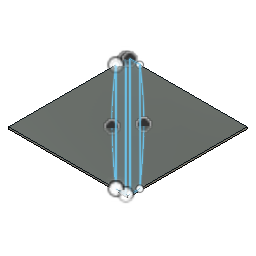
cnc2.2 (Autodesk Fusion 360 design; units mm, degrees)
Autodesk Fusion 360 part; units mm, degrees
sketch "Sketch1" plane through (0, 0, 0) normal (0, 0, 1) x (1, 0, 0)
  line L0 (-120, 100) -> (180, 100)
  line L1 (180, 100) -> (180, -200)
  line L2 (180, -200) -> (-120, -200)
  line L3 (-120, -200) -> (-120, 100)
  dimension "d1" = 300
  dimension "d2" = 300
  constraint perpendicular L0 L1
  constraint parallel L0 L2
  constraint parallel L1 L3
  constraint horizontal L0
  measures "d1" distance of L0.start L0.end
  measures "d2" distance of L0.start L2.end
extrude "Extrude1" add sketch "Sketch1" along normal blind 5
sketch "Sketch2" plane through (0, 0, 0) normal (0, 1, 0) x (1, 0, 0)
sketch "Sketch3" plane through (0, 0, 5) normal (0, 0, 1) x (-1, 0, 0)
  line L0 (120, 200) -> (-180, 200)
  line L1 (-180, 200) -> (-180, -100)
  line L2 (-180, -100) -> (120, -100)
  line L3 (120, -100) -> (120, 200)
  line L4 (120, -95) -> (115, -100)
  line L5 (115, -100) -> (-179.8727, 194.8727)
  line L6 (-179.8727, 194.8727) -> (-174.8727, 199.8727)
  line L7 (-174.8727, 199.8727) -> (120, -95)
  constraint perpendicular L4 L5
  constraint parallel L4 L6
  constraint parallel L5 L7
  constraint coincident L2 L4.end
  constraint coincident L3 L4.start
sketch "Sketch4" plane through (0, 0, 5) normal (0, 0, 1) x (-1, 0, 0)
  line L0 (114.717, -100.0201) -> (89.717, -100.0201)
  dimension "d5" = 25
  constraint horizontal L0
  measures "d5" distance of L0.start L0.end
sketch "Sketch5" plane through (0, 0, 5) normal (0, 0, 1) x (-1, 0, 0)
  line L0 (120.3356, -94.7179) -> (120.3356, -69.7179)
  dimension "d6" = 25
  constraint vertical L0
  measures "d6" distance of L0.start L0.end
sketch "Sketch6" plane through (0, 0, 5) normal (0, 0, 1) x (-1, 0, 0)
  line L0 (-180, 195) -> (-180, 170)
  dimension "d7" = 25
  constraint vertical L0
  measures "d7" distance of L0.start L0.end
sketch "Sketch7" plane through (0, 0, 5) normal (0, 0, 1) x (-1, 0, 0)
  line L0 (-175, 200) -> (-150, 200)
  dimension "d8" = 25
  constraint horizontal L0
  measures "d8" distance of L0.start L0.end
sketch "Sketch8" plane through (0, 0, 5) normal (0, 0, 1) x (-1, 0, 0)
  line L0 (120, -70) -> (-150, 200)
  line L1 (-180.0283, 194.0424) -> (115.3475, -100.2553)
  line L2 (115.3475, -100.2553) -> (90, -100.2553)
  line L3 (90, -100.2553) -> (-180.7976, 169.554)
  line L4 (-180.7976, 169.554) -> (-180.0283, 194.0424)
  constraint horizontal L2
  constraint parallel L1 L3
sketch "Sketch9" plane through (0, 0, 5) normal (0, 0, 1) x (-1, 0, 0)
  line L0 (120.1985, -95.4042) -> (120.1985, -70)
  line L1 (120.1985, -70) -> (-150, 200)
  line L2 (-150, 200) -> (-174.6382, 200)
  line L3 (-174.6382, 200) -> (120.1985, -95.4042)
  constraint vertical L0
  constraint perpendicular L0 L2
sketch "Sketch10" plane through (0, 0, 5) normal (0, 0, 1) x (-1, 0, 0)
  spline S0 degree 5 poles (120, -70) (114.9792, -64.2208) (104.9046, -52.6954) (89.6933, -35.5067) (69.2095, -12.7905) (43.2453, 15.2453) (16.8894, 42.8894) (-9.89, 70.11) (-37.1106, 96.8894) (-64.7547, 123.2453) (-92.7905, 149.2095) (-115.5067, 169.6933) (-132.6954, 184.9046) (-144.2208, 194.9792) (-150, 200) knots 0 0 0 0 0 0 0.1 0.2 0.3 0.4 0.5 0.6 0.7 0.8 0.9 1 1 1 1 1 1
  spline S1 degree 5 poles (90, -100) (84.4105, -95.1738) (73.2481, -85.4708) (56.5546, -70.7647) (34.3984, -50.8484) (6.8843, -25.4047) (-20.433, 0.6347) (-47.5383, 27.3162) (-74.4245, 54.6607) (-101.1019, 82.6371) (-127.587, 111.1957) (-148.6343, 134.4691) (-164.3455, 152.1487) (-174.7872, 164.0332) (-180, 170) knots 0 0 0 0 0 0 0.1 0.2 0.3 0.4 0.5 0.6 0.7 0.8 0.9 1 1 1 1 1 1
  point P0 (-10, 70)
  point P1 (-45, 25)
